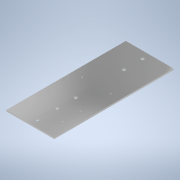
# Autodesk Inventor part: Aluminum Plate
Saved by Autodesk Inventor 2021 (Build 250183000, 183)
## iProperties
Created: 2020-08-21
Part Number: Aluminum Plate
Material: Aluminum 6061
Document SubType Name: Modeling
Designer: Haden
Density: 2.7 g/cm^3
Appearance: Aluminum - Flat
Author: Haden
Autodesk Inventor part; units mm, degrees
ref_plane "YZ Plane" through (0, 0, 0) normal (1, 0, 0) x (0, 1, 0)
ref_plane "XZ Plane" through (0, 0, 0) normal (0, 1, 0) x (-1, 0, 0)
ref_plane "XY Plane" through (0, 0, 0) normal (0, 0, 1) x (1, 0, 0)
sketch "Sketch1" plane through (0, 0, 0) normal (0, 1, 0) x (-1, 0, 0)
  line L0 (0, 0) -> (-100, 0)
  line L1 (-100, 0) -> (-100, -250)
  line L2 (-100, -250) -> (0, -250)
  line L3 (0, -250) -> (0, 0)
  dimension "d0" = 100
  dimension "d1" = 250
  constraints: 8 end point, 2 parallel, 1 horizontal, 1 perpendicular
  measures "d0" distance of L2.end L1.end
  measures "d1" distance of L1.end L0.end
extrude "Extrusion1" add sketch "Sketch1" along normal blind 3
sketch "Sketch2" plane through (0, 3, 0) normal (0, 1, 0) x (1, 0, 0)
  line L0 (0, 0) -> (100, 0) projected
  line L1 (0, 0) -> (20, 38) construction
  line L2 (80, 38) -> (100, 0) construction
  point P0 (20, 75.5)
  point P1 (80, 75.5)
  point P2 (20, 138.5)
  point P3 (80, 138.5)
  dimension "d4" = 60
  dimension "d5" = 37.5
  dimension "d6" = 63
  dimension "d7" = 38
  constraints: 4 end point, 4 vertical alignment, 3 horizontal alignment, 1 equal length
  measures "d4" distance of L2.start L1.end
  measures "d5" distance of point (20, 75.5) L1.end
  measures "d6" distance of point (20, 138.5) point (20, 75.5)
  measures "d7" distance from line of L0 L1.end
hole "Hole1" at (20, 3, -38) at (80, 3, -38) at (20, 3, -75.5) at (80, 3, -75.5) at (20, 3, -138.5) at (80, 3, -138.5) direction (0, -1, 0) diameter 3 end through all
sketch "Sketch3" plane through (0, 3, 0) normal (0, 1, 0) x (1, 0, 0)
  line L0 (0, 0) -> (100, 0) construction
  line L1 (0, 0) -> (50, 15) construction
  line L2 (100, 0) -> (100, 250) construction
  line L3 (50, 15) -> (100, 0) construction
  line L4 (100, 250) -> (0, 250) projected
  point P0 (50, 56.25)
  point P1 (50, 196.204)
  point P2 (50, 95.046)
  point P3 (50, 235)
  dimension "d15" = 15
  dimension "d16" = 41.25
  dimension "d17" = 139.954
  dimension "d25" = 139.954
  dimension "d26" = 15
  constraints: 4 end point, 4 vertical alignment, 1 equal length
  measures "d15" distance from line of L0 L1.end
  measures "d16" distance of L1.end point (50, 56.25)
  measures "d17" distance of point (50, 196.204) point (50, 56.25)
  measures "d25" distance of point (50, 95.046) point (50, 235)
  measures "d26" distance from line of L4 point (50, 235)
hole "Hole2" at (50, 3, -15) at (50, 3, -56.25) at (50, 3, -196.204) at (50, 3, -95.046) at (50, 3, -235) direction (0, -1, 0) diameter 6.35 end through all
equation "\"d25\" = d17"
body "Solid1"
